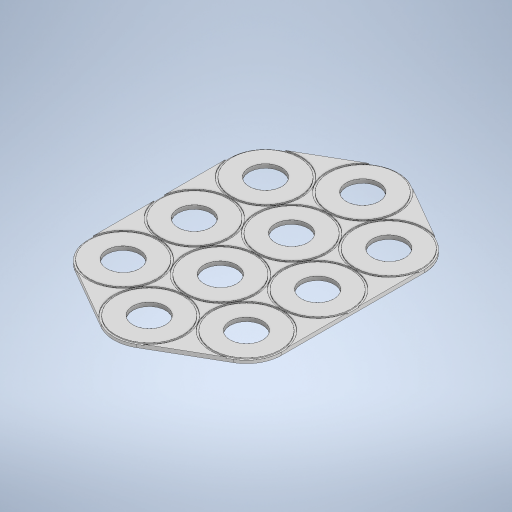
# Autodesk Inventor part: Separador_10_amostras_v2
Saved by Autodesk Inventor 2024 (Build 280153000, 153)
## iProperties
Created: 2025-07-22
Part Number: Separador_10_amostras_v2
Material: Generic
Document SubType Name: Modeling
Designer: Bruno
Density: 1 g/cm^3
Appearance: Default
Author: Bruno
Autodesk Inventor part; units mm, degrees
ref_plane "YZ Plane" through (0, 0, 0) normal (1, 0, 0) x (0, 1, 0)
ref_plane "XZ Plane" through (0, 0, 0) normal (0, 1, 0) x (-1, 0, 0)
ref_plane "XY Plane" through (0, 0, 0) normal (0, 0, 1) x (1, 0, 0)
sketch "Sketch1" plane through (0, 0, 0) normal (0, 1, 0) x (-1, 0, 0)
  line L0 (100, -100) -> (-100, -100)
  line L1 (-100, -100) -> (-100, 100)
  line L2 (-100, 100) -> (100, 100)
  line L3 (100, 100) -> (100, -100)
  line L4 (100, -100) -> (-100, 100)
  point P0 (0, 0)
  point P1 (0, 0)
  dimension "d0" = 200
  dimension "d1" = 200
  constraints: 10 end point, 2 parallel, 1 coincident, 1 horizontal, 1 midpoint, 1 perpendicular
  measures "d0" distance of L0.end L1.end
  measures "d1" distance of L0.start L0.end
extrude "Extrusion1" add sketch "Sketch1" along normal blind 2
sketch "Sketch2" plane through (0, 2, 0) normal (0, 1, 0) x (1, 0, 0)
  line L0 (100, 100) -> (-100, 100) projected
  line L1 (0, 100) -> (0, -100)
  line L2 (-100, -100) -> (100, -100) projected
  line L3 (100, -100) -> (100, 100) projected
  line L4 (100, 0) -> (-100, 0)
  line L5 (-100, 100) -> (-100, -100) projected
  circle A0 centre (0, -55.5) radius 18.5
  circle A1 centre (0, -55.5) radius 8.5
  circle A2 centre (0, -55.5) radius 17.5
  circle A3 centre (0, -55.5) radius 7.5
  circle A4 centre (0, -18.5) radius 7.5
  circle A5 centre (0, -18.5) radius 8.5
  circle A6 centre (0, -18.5) radius 17.5
  circle A7 centre (0, -18.5) radius 18.5
  circle A8 centre (0, 18.5) radius 7.5
  circle A9 centre (0, 18.5) radius 8.5
  circle A10 centre (0, 18.5) radius 17.5
  circle A11 centre (0, 18.5) radius 18.5
  circle A12 centre (0, 55.5) radius 7.5
  circle A13 centre (0, 55.5) radius 8.5
  circle A14 centre (0, 55.5) radius 17.5
  circle A15 centre (0, 55.5) radius 18.5
  circle A16 centre (-32.0429, -37) radius 7.5
  circle A17 centre (-32.0429, -37) radius 8.5
  circle A18 centre (-32.0429, -37) radius 17.5
  circle A19 centre (-32.0429, -37) radius 18.5
  circle A20 centre (-32.0429, 0) radius 7.5
  circle A21 centre (-32.0429, 0) radius 8.5
  circle A22 centre (-32.0429, 0) radius 17.5
  circle A23 centre (-32.0429, 0) radius 18.5
  circle A24 centre (-32.0429, 37) radius 7.5
  circle A25 centre (-32.0429, 37) radius 8.5
  circle A26 centre (-32.0429, 37) radius 17.5
  circle A27 centre (-32.0429, 37) radius 18.5
  circle A28 centre (32.0571, -37) radius 7.5
  circle A29 centre (32.0571, -37) radius 8.5
  circle A30 centre (32.0571, -37) radius 17.5
  circle A31 centre (32.0571, -37) radius 18.5
  circle A32 centre (32.0571, 0) radius 7.5
  circle A33 centre (32.0571, 0) radius 8.5
  circle A34 centre (32.0571, 0) radius 17.5
  circle A35 centre (32.0571, 0) radius 18.5
  circle A36 centre (32.0571, 37) radius 7.5
  circle A37 centre (32.0571, 37) radius 8.5
  circle A38 centre (32.0571, 37) radius 17.5
  circle A39 centre (32.0571, 37) radius 18.5
  point P0 (0, 0)
  point P1 (-32.0429, 18.5)
  point P2 (-16.0215, 27.75)
  point P3 (-16.0215, 46.25)
  point P4 (-16.0215, 9.25)
  point P5 (-32.0429, -18.5)
  point P6 (-16.0215, -9.25)
  point P7 (0, 37)
  point P8 (0, 0)
  point P9 (-16.0215, -27.75)
  point P10 (32.0571, 18.5)
  point P11 (32.0571, -18.5)
  dimension "d4" = 37
  dimension "d5" = 17
  dimension "d18" = 35
  dimension "d19" = 15
  dimension "d42" = 37
  dimension "d47" = 111
  dimension "d48" = 35
  dimension "d49" = 37
  dimension "d50" = 15
  dimension "d51" = 17
  dimension "d55" = 37
  dimension "d58" = 64.1
  constraints: 40 centre point, 30 coincident, 4 end point, 4 midpoint, 2 equal radius, 2 vertical, 1 horizontal, 1 point on line, 64 other
  measures "d4" diameter of A0
  measures "d5" diameter of A1
  measures "d18" diameter of A2
  measures "d19" diameter of A3
  measures "d42" distance of A3.centre A4.centre
  measures "d47" diameter of A0.centre L4
  measures "d48" diameter of A18
  measures "d49" diameter of A19
  measures "d50" diameter of A16
  measures "d51" diameter of A17
  measures "d55" distance of A16.centre A20.centre
  measures "d58" distance of A16.centre A28.centre
extrude "Extrusion2" cut sketch "Sketch2" against normal blind 0.5 contours A39 | A31 | A15 L1 A14 | L1 A14 A15 | A35 L4 A34 | L4 A34 A35 | A27 | A23 L4 A22 | L4 A22 A23 | A13 L1 A12 | L1 A12 A13 | A11 L1 A10 | L1 A10 A11 | A0 L1 A2 | L1 A2 A0 | A33 L4 A32 | L4 A32 A33 | A19 | A7 L1 A6 | L1 A6 A7 | A21 L4 A20 | L4 A20 A21 | A9 L1 A8 | L1 A8 A9 | A1 L1 A3 | L1 A3 A1 | A5 L1 A4 | L1 A4 A5 | A17 | A25 | A29 | A37
sketch "Sketch4" plane through (0, 2, 0) normal (0, 1, 0) x (1, 0, 0)
  arc A0 (-16.0215, 46.25) -> (-32.0429, 18.5) centre (-32.0429, 37) ccw projected
  line L0 (-41.2929, 53.0215) -> (-9.25, 71.5215)
  arc A1 (0, 37) -> (-16.0215, 46.25) centre (0, 55.5) ccw projected
  line L1 (9.2469, 71.5232) -> (41.304, 53.0232)
  circle A2 centre (32.0571, 37) radius 18.5 projected
  line L2 (50.5571, 37) -> (50.5571, -37)
  circle A3 centre (32.0571, -37) radius 18.5 projected
  line L3 (41.304, -53.0232) -> (9.2469, -71.5232)
  arc A4 (-16.0215, -46.25) -> (0, -37) centre (0, -55.5) ccw projected
  line L4 (-9.25, -71.5215) -> (-41.2929, -53.0215)
  line L5 (-50.5429, 37) -> (-50.5429, -37)
  arc A5 (-32.0429, -18.5) -> (-16.0215, -46.25) centre (-32.0429, -37) ccw projected
  line L6 (-100, 100) -> (-100, -100) projected
  line L7 (100, 100) -> (-100, 100) projected
  line L8 (100, -100) -> (100, 100) projected
  line L9 (-100, -100) -> (100, -100) projected
  point P0 (0, 0)
  point P1 (32.0571, 18.5)
  point P2 (32.0571, -18.5)
  constraints: 12 end point, 12 point on circle, 12 tangent
extrude "Extrusion4" cut sketch "Sketch4" against normal through all
sketch "Sketch5" plane through (0, 2, -18.5) normal (0, 1, 0) x (1, 0, 0)
  circle A0 centre (-32.0429, 18.5) radius 8.5 projected
  circle A1 centre (0, 37) radius 8.5 projected
  circle A2 centre (32.0571, 18.5) radius 8.5 projected
  circle A3 centre (0, 0) radius 8.5 projected
  circle A4 centre (32.0571, -18.5) radius 8.5 projected
  circle A5 centre (32.0571, -55.5) radius 8.5 projected
  circle A6 centre (0, -37) radius 8.5 projected
  circle A7 centre (0, -74) radius 8.5 projected
  circle A8 centre (-32.0429, -55.5) radius 8.5 projected
  circle A9 centre (-32.0429, -18.5) radius 8.5 projected
  arc A10 (41.304, -71.5232) -> (50.5571, -55.5) centre (32.0571, -55.5) ccw projected
  line L0 (41.304, -71.5232) -> (9.2469, -90.0232) projected
  arc A11 (-9.25, -90.0215) -> (9.2469, -90.0232) centre (0, -74) ccw projected
  line L1 (-9.25, -90.0215) -> (-41.2929, -71.5215) projected
  arc A12 (-50.5429, -55.5) -> (-41.2929, -71.5215) centre (-32.0429, -55.5) ccw projected
  line L2 (-50.5429, -55.5) -> (-50.5429, 18.5) projected
  arc A13 (-41.2929, 34.5215) -> (-50.5429, 18.5) centre (-32.0429, 18.5) ccw projected
  line L3 (-41.2929, 34.5215) -> (-9.25, 53.0215) projected
  arc A14 (9.2469, 53.0232) -> (-9.25, 53.0215) centre (0, 37) ccw projected
  line L4 (9.2469, 53.0232) -> (41.304, 34.5232) projected
  arc A15 (50.5571, 18.5) -> (41.304, 34.5232) centre (32.0571, 18.5) ccw projected
  line L5 (50.5571, 18.5) -> (50.5571, -55.5) projected
  line L6 (41.204, 34.35) -> (9.147, 52.85)
  arc A16 (9.147, 52.85) -> (-9.15, 52.8483) centre (0, 37) ccw
  line L7 (-9.15, 52.8483) -> (-41.1929, 34.3483)
  arc A17 (-41.1929, 34.3483) -> (-50.3429, 18.5) centre (-32.0429, 18.5) ccw
  line L8 (-50.3429, 18.5) -> (-50.3429, -55.5)
  arc A18 (-50.3429, -55.5) -> (-41.1929, -71.3483) centre (-32.0429, -55.5) ccw
  line L9 (-41.1929, -71.3483) -> (-9.15, -89.8483)
  arc A19 (-9.15, -89.8483) -> (9.147, -89.85) centre (0, -74) ccw
  line L10 (9.147, -89.85) -> (41.204, -71.35)
  arc A20 (41.204, -71.35) -> (50.3571, -55.5) centre (32.0571, -55.5) ccw
  line L11 (50.3571, -55.5) -> (50.3571, 18.5)
  arc A21 (50.3571, 18.5) -> (41.204, 34.35) centre (32.0571, 18.5) ccw
  point P0 (0, -18.5)
  dimension "d65" = 0.2
  constraints: 12 end point, 12 point on circle, 6 centre point, 11 other
  measures "d65" distance between parallel lines of L4 L6
extrude "Extrusion5" cut sketch "Sketch5" against normal through all
body "Solid1"
